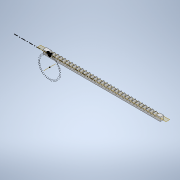
# Autodesk Inventor part: Rack
Saved by Autodesk Inventor 2020 (Build 240168000, 168)
## iProperties
Created: 2021-01-11
Part Number: Rack
Material: Generic
Document SubType Name: Modeling
Designer: moham
Density: 1 g/cm^3
Appearance: Default
Author: moham
Autodesk Inventor part; units mm, degrees
ref_plane "YZ Plane" through (0, 0, 0) normal (1, 0, 0) x (0, 1, 0)
ref_plane "XY Plane" through (0, 0, 0) normal (0, 0, 1) x (1, 0, 0)
sketch "Sketch4" plane through (0, 0, 0) normal (0, 0, 1) x (1, 0, 0)
  line L0 (-11.7536, 21.827) -> (198.2464, 21.827)
  line L1 (198.2464, 21.827) -> (198.2464, 14.827)
  line L2 (198.2464, 14.827) -> (-11.7536, 14.827)
  line L3 (-11.7536, 14.827) -> (-11.7536, 21.827)
  point P0 (0, 0)
  point P1 (-2.7536, 21.827)
  point P2 (2.7536, 21.827)
  dimension "d9" = 210
  dimension "d10" = 7
  dimension "d11" = 9
  constraints: 8 end point, 2 parallel, 1 horizontal, 1 perpendicular, 1 point on line
  measures "d9" distance of L1.end L2.end
  measures "d10" distance of L0.end L1.end
  measures "d11" distance from line of point (-2.754, 21.827) L3
sketch "Sketch1" plane through (0, 0, 0) normal (0, 0, 1) x (1, 0, 0)
  spline S0 degree 3 poles (-2.7536, 21.827) (-2.6838, 21.738) (-2.5443, 21.5601) (-2.346, 21.2847) (-2.1563, 21.0035) (-1.9767, 20.7156) (-1.8081, 20.4212) (-1.6519, 20.12) (-1.5096, 19.8119) (-1.3837, 19.4968) (-1.2951, 19.2281) (-1.2382, 19.0093) (-1.2032, 18.8431) (-1.1864, 18.6741) (-1.1548, 18.5074) (-1.1137, 18.3427) (-1.0578, 18.1823) (-0.9848, 18.0289) (-0.8938, 17.8852) (-0.8001, 17.7787) (-0.7163, 17.7026) (-0.6476, 17.6528) (-0.5762, 17.6068) (-0.4992, 17.5709) (-0.4204, 17.5391) (-0.3379, 17.5188) (-0.2545, 17.503) (-0.1413, 17.4982) (0, 17.5012) (0.1413, 17.4982) (0.2545, 17.503) (0.3379, 17.5188) (0.4204, 17.5391) (0.4992, 17.5709) (0.5762, 17.6068) (0.6476, 17.6528) (0.7163, 17.7026) (0.8001, 17.7787) (0.8938, 17.8852) (0.9848, 18.0289) (1.0578, 18.1823) (1.1137, 18.3427) (1.1548, 18.5074) (1.1864, 18.6741) (1.2032, 18.8431) (1.2382, 19.0093) (1.2951, 19.2281) (1.3837, 19.4968) (1.5096, 19.8119) (1.6519, 20.12) (1.8081, 20.4212) (1.9767, 20.7156) (2.1563, 21.0035) (2.346, 21.2847) (2.5443, 21.5601) (2.6838, 21.738) (2.7536, 21.827) knots 0 0 0 0 0.03392 0.067841 0.101761 0.135682 0.169602 0.203521 0.23744 0.271357 0.305272 0.322231 0.339189 0.356149 0.373109 0.390064 0.407022 0.423978 0.44093 0.457876 0.466358 0.474834 0.483315 0.491794 0.500274 0.508752 0.517232 0.52571 0.54267 0.559631 0.568109 0.576589 0.585067 0.593547 0.602026 0.610507 0.618983 0.627465 0.644411 0.661363 0.678319 0.695277 0.712232 0.729192 0.746152 0.763109 0.780069 0.813984 0.847901 0.88182 0.915739 0.949659 0.98358 1.0175 1.051421 1.085341 1.085341 1.085341 1.085341
  circle A0 centre (0, 0) radius 17.5 construction
  circle A1 centre (0, 0) radius 18.7939 construction
  circle A2 centre (0, 0) radius 20 construction
  line L0 (-2.7536, 21.827) -> (2.7536, 21.827)
  line L1 (-64, 20) -> (85, 20)
  point P0 (-2.5461, 21.5587)
  point P1 (-2.3474, 21.2837)
  point P2 (-2.158, 21.0024)
  point P3 (-1.9785, 20.7145)
  point P4 (-1.8102, 20.42)
  point P5 (-1.6542, 20.1188)
  point P6 (-1.5123, 19.8107)
  point P7 (-1.387, 19.4956)
  point P8 (-1.2821, 19.1731)
  point P9 (-1.2395, 19.0089)
  point P10 (-1.2062, 18.8426)
  point P11 (-1.1839, 18.6745)
  point P12 (-1.1532, 18.5077)
  point P13 (-1.1112, 18.3434)
  point P14 (-1.0549, 18.1835)
  point P15 (-0.9818, 18.0305)
  point P16 (-0.8902, 17.8878)
  point P17 (-0.7784, 17.7605)
  point P18 (-0.7153, 17.7038)
  point P19 (-0.6471, 17.6535)
  point P20 (-0.5752, 17.6085)
  point P21 (-0.4989, 17.5716)
  point P22 (-0.4198, 17.541)
  point P23 (-0.3378, 17.5195)
  point P24 (-0.2542, 17.505)
  point P25 (-0.1696, 17.5)
  point P26 (0, 17.5)
  point P27 (0.1696, 17.5)
  point P28 (0.2542, 17.505)
  point P29 (0.3378, 17.5195)
  point P30 (0.4198, 17.541)
  point P31 (0.4989, 17.5716)
  point P32 (0.5752, 17.6085)
  point P33 (0.6471, 17.6535)
  point P34 (0.7153, 17.7038)
  point P35 (0.7784, 17.7605)
  point P36 (0.8902, 17.8878)
  point P37 (0.9818, 18.0305)
  point P38 (1.0549, 18.1835)
  point P39 (1.1112, 18.3434)
  point P40 (1.1532, 18.5077)
  point P41 (1.1839, 18.6745)
  point P42 (1.2062, 18.8426)
  point P43 (1.2395, 19.0089)
  point P44 (1.2821, 19.1731)
  point P45 (1.387, 19.4956)
  point P46 (1.5123, 19.8107)
  point P47 (1.6542, 20.1188)
  point P48 (1.8102, 20.42)
  point P49 (1.9785, 20.7145)
  point P50 (2.158, 21.0024)
  point P51 (2.3474, 21.2837)
  point P52 (2.5461, 21.5587)
  constraints: 4 end point, 3 centre point, 3 horizontal, 1 tangent, 114 other
pattern_of_nothing "Circular Pattern1"
extrude "Extrusion3" add sketch "Sketch4" against normal blind 6
extrude "Extrusion4" cut sketch "Sketch1" against normal blind 6
pattern_linear "Rectangular Pattern1" count 31 spacing 6.2832 along (1, 0, 0) of "Extrusion4"
ref_plane "Work Plane1" through (-64, 20, 0) normal (0, 1, 0) x (-1, 0, 0)
equation "\"Module\" = 2"
equation "\"PressureAngle\" = 20deg"
equation "\"UnitProfileClearance\" = 0.25"
equation "\"UnitRoundRadius\" = 0.35"
equation "\"HeadDiameter\" = 44"
equation "\"RootDiameter\" = 35"
equation "\"BaseDiameter\" = 37.5877"
equation "\"FaceWidth\" = 6"
equation "\"HelixAngle\" = 0"
equation "\"UnitCorrection\" = 0"
equation "\"UnitAddendumModification\" = 0"
equation "\"CircularPitch\" = 6.283185"
equation "\"UnitBacklashShift\" = 0"
equation "\"TotalToolShift\" = 0"
equation "\"IsInternal\" = 0"
body "Solid2"
